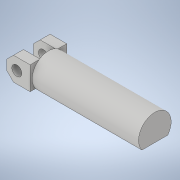
# Autodesk Inventor part: Hammer
Saved by Autodesk Inventor 2021 (Build 250183000, 183)
## iProperties
Created: 2021-03-07
Part Number: Hammer
Material: Generic
Document SubType Name: Modeling
Designer: Lukas
Density: 1 g/cm^3
Appearance: Default
Author: Lukas
Autodesk Inventor part; units mm, degrees
ref_plane "YZ Plane" through (0, 0, 0) normal (1, 0, 0) x (0, 1, 0)
ref_plane "XZ Plane" through (0, 0, 0) normal (0, 1, 0) x (-1, 0, 0)
ref_plane "XY Plane" through (0, 0, 0) normal (0, 0, 1) x (1, 0, 0)
sketch "Sketch5" plane through (0, 0, 0) normal (0, 0, 1) x (1, 0, 0)
  line L0 (-32, 0) -> (0, 0)
  line L1 (0, 4.9) -> (0, 0)
  line L2 (-32, 4.9) -> (0, 4.9)
  line L3 (-32, 4.9) -> (-32, 0)
  dimension "d95" = 4.9
  dimension "d106" = 32
  constraints: 8 end point, 2 horizontal, 2 vertical
  measures "d95" distance of L1.start L0.end
  measures "d106" distance of L2.start L1.start
revolve "Revolution1" add sketch "Sketch5" angle 360 about axis through (-32, 0, 0) along (1, 0, 0)
sketch "Sketch6" plane through (0, 0, 0) normal (1, 0, 0) x (0, 0, -1)
  circle A0 centre (0, 0) radius 4.9 projected
  circle A1 centre (0, 0) radius 4.9 projected
  line L0 (-3.8743, -3) -> (3.8743, -3)
  dimension "d96" = 3
  constraints: 2 end point, 2 point on circle, 1 horizontal
  measures "d96" distance from line of point (0, 0) L0
extrude "Extrusion5" cut sketch "Sketch6" against normal blind 53 contours L0 A0 picked at (-1.032, -3.266)
sketch "Sketch7" plane through (-32, 0, 0) normal (-1, 0, 0) x (0, 0, 1)
  line L0 (-2.5, 4) -> (-5.5, 4)
  line L1 (-5.5, 4) -> (-5.5, -3)
  line L2 (-5.5, -3) -> (-2.5, -3)
  line L3 (-2.5, -3) -> (-2.5, 4)
  line L4 (2.5, -3) -> (5.5, -3)
  line L5 (5.5, -3) -> (5.5, 4)
  line L6 (5.5, 4) -> (2.5, 4)
  line L7 (2.5, 4) -> (2.5, -3)
  point P0 (0, 0)
  dimension "d111" = 5
  dimension "d112" = 2.5
  dimension "d113" = 3
  dimension "d114" = 4
  dimension "d115" = 3
  constraints: 16 end point, 4 parallel, 2 equal length, 2 horizontal, 2 perpendicular, 1 point on line
  measures "d111" distance between parallel lines of L7 L3
  measures "d112" distance from line of L3 point (0, 0)
  measures "d113" distance from line of point (0, 0) L2
  measures "d114" distance from line of point (0, 0) L0
  measures "d115" distance of L0.start L0.end
extrude "Extrusion6" add sketch "Sketch7" along normal blind 7
sketch "Sketch9" plane through (-32, -2.8284, 5.5) normal (0, 0, 1) x (1, 0, 0)
  circle A0 centre (-4, 3.3284) radius 1.5
  line L0 (0, -0.1716) -> (0, 6.8284) projected
  point P0 (32, 2.8284)
  point P1 (0, 3.3284)
  dimension "d108" = 3
  dimension "d116" = 4
  constraints: 1 centre point, 1 horizontal alignment, 1 midpoint
  measures "d108" diameter of A0
  measures "d116" distance from line of L0 A0.centre
extrude "Extrusion8" cut sketch "Sketch9" against normal through all
chamfer "Chamfer2" [suppressed]
chamfer "Chamfer3" distance 3.5 distance2 2 1 edges at (-32, -3, 0) measured on face at (-32, -2.5, 0)
chamfer "Chamfer4" distance 2 angle 45 4 edges at (-39, 4, -4) (-39, 4, 4) (-39, -3, -4) (-39, -3, 4)
body "Solid2"
